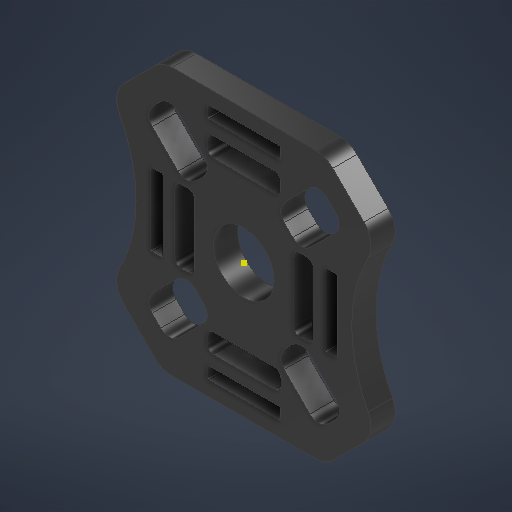
# Autodesk Inventor part: atasandrone
Saved by Autodesk Inventor 2026.1 (Build 301233000, 233)
## iProperties
Created: 2026-03-03
Part Number: atasandrone
Material: Generic
Document SubType Name: Modeling
Designer: ayjuni03
Density: 1 g/cm^3
Appearance: Default
Author: ayjuni03
Autodesk Inventor part; units mm, degrees
ref_plane "YZ Plane" through (0, 0, 0) normal (1, 0, 0) x (0, 1, 0)
ref_plane "XZ Plane" through (0, 0, 0) normal (0, 1, 0) x (-1, 0, 0)
ref_plane "XY Plane" through (0, 0, 0) normal (0, 0, 1) x (1, 0, 0)
sketch "Sketch1" plane through (0, 0, 0) normal (0, 0, 1) x (1, 0, 0)
  line L0 (0, 0) -> (55, 0)
  line L1 (55, 0) -> (-55, 0)
  line L2 (-55, 0) -> (-55, 55)
  line L3 (-55, 33.743) -> (-55, -33.7433)
  line L4 (-29.6762, -55) -> (29.5764, -55)
  line L5 (-29.5258, 55) -> (29.5764, 55)
  line L6 (55.0505, 33.743) -> (55.0505, -33.7433)
  line L7 (-49.4757, -39.2903) -> (-36.7617, -52.0566) construction
  line L8 (-49.4757, -39.2903) -> (-36.7617, -52.0566)
  line L9 (-55, -33.7433) -> (55.0505, -33.7433) construction
  line L10 (-55, -55) -> (-33.8303, -55) construction
  line L11 (55.0505, -55) -> (33.7065, -55) construction
  line L12 (36.633, -52.0856) -> (49.4815, -39.2896)
  line L13 (-55, -55) -> (-55, -33.7433) construction
  line L14 (-55, -55) -> (-55, -33.7433) construction
  line L15 (-55, -33.7433) -> (-55, -55) construction
  line L16 (-55, -33.7433) -> (-55, -55) construction
  line L17 (-55, 55) -> (-55, 33.743) construction
  line L18 (-55, 55) -> (-33.656, 55) construction
  line L19 (-36.5824, 52.0855) -> (-49.4311, 39.2892)
  line L20 (55.0505, 55) -> (47.34, 55) construction
  line L21 (33.7065, 55) -> (55.0505, 55) construction
  line L22 (55.0505, 55) -> (55.0505, 33.743) construction
  line L23 (49.4816, 39.2892) -> (36.633, 52.0855)
  arc A0 (-51.2319, -27.5622) -> (-51.2185, 27.5365) centre (-103.3983, -0.0002) ccw
  arc A1 (51.2691, 27.5365) -> (51.269, -27.5368) centre (103.4489, -0.0002) ccw
  arc A2 (-49.4311, 39.2892) -> (-51.2185, 27.5365) centre (-42.3745, 32.2037) ccw
  arc A3 (-29.5258, 55) -> (-36.5824, 52.0855) centre (-29.5258, 45) ccw
  arc A4 (36.633, 52.0855) -> (29.5764, 55) centre (29.5764, 45) ccw
  arc A5 (51.2691, 27.5365) -> (49.4816, 39.2892) centre (42.425, 32.2037) ccw
  arc A6 (49.4815, -39.2896) -> (51.269, -27.5368) centre (42.425, -32.204) ccw
  arc A7 (29.5764, -55) -> (36.633, -52.0856) centre (29.5764, -45) ccw
  arc A8 (-36.7617, -52.0566) -> (-29.6762, -55) centre (-29.6762, -45) ccw
  arc A9 (-51.2319, -27.5622) -> (-49.4757, -39.2903) centre (-42.3902, -32.2338) ccw
  line L24 (-0.0499, -55) -> (-0.0499, -49) construction
  line L25 (-0.0499, -49) -> (14.4501, -49)
  line L26 (14.9501, -49) -> (-14.5499, -49)
  line L27 (-15.0499, -48.5) -> (-15.0499, -44.5)
  line L28 (-14.5499, -44) -> (14.4501, -44)
  line L29 (14.9501, -44.5) -> (14.9501, -48.5)
  arc A10 (14.4501, -49) -> (14.9501, -48.5) centre (14.4501, -48.5) ccw
  arc A11 (14.9501, -44.5) -> (14.4501, -44) centre (14.4501, -44.5) ccw
  arc A12 (-14.5499, -44) -> (-15.0499, -44.5) centre (-14.5499, -44.5) ccw
  arc A13 (-15.0499, -48.5) -> (-14.5499, -49) centre (-14.5499, -48.5) ccw
  line L30 (-36.0332, -38.6169) -> (-43.1187, -45.6734) construction
  line L31 (-36.0332, -38.6169) -> (-34.269, -40.3883) construction
  line L32 (-34.269, -40.3883) -> (-37.7973, -36.8455) construction
  line L33 (-37.7828, -29.7744) -> (-27.1545, -19.1896) construction
  line L34 (-20.0834, -19.2041) -> (-16.5552, -22.7469) construction
  line L35 (-16.5697, -29.8179) -> (-27.198, -40.4028) construction
  line L36 (-16.5697, -29.8179) -> (-27.198, -40.4028)
  line L37 (-37.7828, -29.7744) -> (-23.6117, -15.6613)
  line L38 (-16.5552, -22.7469) -> (-20.0834, -19.2041)
  arc A14 (-37.7828, -29.7744) -> (-37.7973, -36.8455) centre (-34.2545, -33.3172) ccw
  arc A15 (-34.269, -40.3883) -> (-27.198, -40.4028) centre (-30.7263, -36.86) ccw
  arc A16 (-16.5697, -29.8179) -> (-16.5552, -22.7469) centre (-20.0979, -26.2752) ccw
  arc A17 (-20.0834, -19.2041) -> (-27.1545, -19.1896) centre (-23.6262, -22.7324) ccw
  line L39 (-41.3256, -33.3027) -> (-40.8868, -33.7433)
  line L40 (-37.7973, -36.8455) -> (-34.269, -40.3883)
  line L41 (-42.3902, -32.2338) -> (-34.269, -40.3883) construction
  line L42 (-30.7408, -43.931) -> (-29.6762, -45) construction
  line L43 (-43.1187, -45.6734) -> (43.0572, -45.6876) construction
  line L44 (43.0572, -45.6876) -> (36.0007, -38.602) construction
  line L45 (36.0007, -38.602) -> (37.7721, -36.8379) construction
  line L46 (27.1583, -40.3516) -> (16.5734, -29.7233) construction
  line L47 (13.0451, -26.1805) -> (20.1307, -19.124) construction
  line L48 (27.2017, -19.1385) -> (37.7866, -29.7668) construction
  line L49 (20.1307, -19.124) -> (16.5879, -22.6523)
  line L50 (27.1583, -40.3516) -> (16.5734, -29.7233)
  line L51 (27.2017, -19.1385) -> (37.7866, -29.7668)
  arc A18 (27.2017, -19.1385) -> (20.1307, -19.124) centre (23.659, -22.6668) ccw
  arc A19 (16.5879, -22.6523) -> (16.5734, -29.7233) centre (20.1162, -26.195) ccw
  arc A20 (37.7721, -36.8379) -> (37.7866, -29.7668) centre (34.2438, -33.2951) ccw
  line L52 (41.3149, -33.3096) -> (40.8793, -33.7433) construction
  line L53 (37.7721, -36.8379) -> (34.2293, -40.3661) construction
  line L54 (30.6865, -43.8944) -> (37.7721, -36.8379) construction
  line L55 (40.8793, -33.7433) -> (41.3149, -33.3096) construction
  line L56 (42.425, -32.204) -> (40.8793, -33.7433) construction
  line L57 (37.7721, -36.8379) -> (29.5764, -45) construction
  line L58 (41.3149, -33.3096) -> (40.8793, -33.7433)
  line L59 (37.7721, -36.8379) -> (34.2293, -40.3661)
  arc A21 (27.1583, -40.3516) -> (34.2293, -40.3661) centre (30.701, -36.8234) ccw
  circle A22 centre (0, 0) radius 12.5
  line L60 (-0.0499, -44) -> (-0.0499, -39) construction
  line L61 (-0.0499, -39) -> (12.6162, -39) construction
  line L62 (12.6162, -39) -> (-0.0499, -39)
  line L63 (-0.0499, -39) -> (-12.5979, -39)
  line L64 (-15.0979, -36.5) -> (-15.0979, -33.5)
  line L65 (-12.5979, -31) -> (12.6162, -31)
  line L66 (15.1162, -33.5) -> (15.1162, -36.5)
  arc A23 (15.1162, -33.5) -> (12.6162, -31) centre (12.6162, -33.5) ccw
  arc A24 (12.6162, -39) -> (15.1162, -36.5) centre (12.6162, -36.5) ccw
  arc A25 (-12.5979, -31) -> (-15.0979, -33.5) centre (-12.5979, -33.5) ccw
  arc A26 (-15.0979, -36.5) -> (-12.5979, -39) centre (-12.5979, -36.5) ccw
  line L67 (-44.3983, -0.0145) -> (-38.3983, 0) construction
  line L68 (44.4489, -0.0001) -> (38.4489, 0) construction
  line L69 (-38.3983, 0) -> (-38.3983, 14.5)
  line L70 (-38.3983, 15) -> (-38.3983, -14.5)
  line L71 (-37.8983, -15) -> (-33.8983, -15)
  line L72 (-33.3983, -14.5) -> (-33.3983, 14.5)
  line L73 (-33.8983, 15) -> (-37.8983, 15)
  arc A27 (-33.3983, 14.5) -> (-33.8983, 15) centre (-33.8983, 14.5) ccw
  arc A28 (-37.8983, 15) -> (-38.3983, 14.5) centre (-37.8983, 14.5) ccw
  arc A29 (-38.3983, -14.5) -> (-37.8983, -15) centre (-37.8983, -14.5) ccw
  arc A30 (-33.8983, -15) -> (-33.3983, -14.5) centre (-33.8983, -14.5) ccw
  line L74 (-33.3983, 0) -> (-28.3983, 0) construction
  line L75 (-28.3983, 0) -> (-28.3983, 12.5)
  line L76 (-28.3983, 12.5) -> (-28.3983, -12.5)
  line L77 (-25.8983, -15) -> (-22.8983, -15)
  line L78 (-20.3983, -12.5) -> (-20.3983, 12.5)
  line L79 (-22.8983, 15) -> (-25.8983, 15)
  arc A31 (-20.3983, 12.5) -> (-22.8983, 15) centre (-22.8983, 12.5) ccw
  arc A32 (-25.8983, 15) -> (-28.3983, 12.5) centre (-25.8983, 12.5) ccw
  arc A33 (-28.3983, -12.5) -> (-25.8983, -15) centre (-25.8983, -12.5) ccw
  arc A34 (-22.8983, -15) -> (-20.3983, -12.5) centre (-22.8983, -12.5) ccw
  line L80 (38.4489, 0) -> (38.4489, -14.5)
  line L81 (38.4489, -15) -> (38.4489, 14.5)
  line L82 (37.9489, 15) -> (33.9489, 15)
  line L83 (33.4489, 14.5) -> (33.4489, -14.5)
  line L84 (33.9489, -15) -> (37.9489, -15)
  arc A35 (38.4489, 14.5) -> (37.9489, 15) centre (37.9489, 14.5) ccw
  arc A36 (33.9489, 15) -> (33.4489, 14.5) centre (33.9489, 14.5) ccw
  arc A37 (33.4489, -14.5) -> (33.9489, -15) centre (33.9489, -14.5) ccw
  arc A38 (37.9489, -15) -> (38.4489, -14.5) centre (37.9489, -14.5) ccw
  line L85 (33.4489, 0) -> (28.4489, 0) construction
  line L86 (28.4489, 0) -> (28.4489, 12.5)
  line L87 (28.4489, 15) -> (28.4489, -12.5)
  line L88 (25.9489, -15) -> (22.9489, -15)
  line L89 (20.4489, -12.5) -> (20.4489, 12.5)
  line L90 (22.9489, 15) -> (25.9489, 15)
  arc A39 (28.4489, 12.5) -> (25.9489, 15) centre (25.9489, 12.5) ccw
  arc A40 (22.9489, 15) -> (20.4489, 12.5) centre (22.9489, 12.5) ccw
  arc A41 (20.4489, -12.5) -> (22.9489, -15) centre (22.9489, -12.5) ccw
  arc A42 (25.9489, -15) -> (28.4489, -12.5) centre (25.9489, -12.5) ccw
  line L91 (0.0253, 55) -> (0.0253, 49) construction
  line L92 (0.0253, 49) -> (14.5253, 49)
  line L93 (15.0253, 49) -> (-14.4747, 49)
  line L94 (-14.9747, 48.5) -> (-14.9747, 44.5)
  line L95 (-14.4747, 44) -> (14.5253, 44)
  line L96 (15.0253, 44.5) -> (15.0253, 48.5)
  arc A43 (15.0253, 48.5) -> (14.5253, 49) centre (14.5253, 48.5) ccw
  arc A44 (14.5253, 44) -> (15.0253, 44.5) centre (14.5253, 44.5) ccw
  arc A45 (-14.9747, 44.5) -> (-14.4747, 44) centre (-14.4747, 44.5) ccw
  arc A46 (-14.4747, 49) -> (-14.9747, 48.5) centre (-14.4747, 48.5) ccw
  line L97 (0.0253, 44) -> (0.0253, 39) construction
  line L98 (0.0253, 39) -> (12.5253, 39)
  line L99 (15.0253, 36.5) -> (15.0253, 33.5)
  line L100 (12.5253, 31) -> (-12.4747, 31)
  line L101 (-14.9747, 33.5) -> (-14.9747, 36.5)
  line L102 (-12.4747, 39) -> (0.0253, 39)
  arc A47 (-12.4747, 39) -> (-14.9747, 36.5) centre (-12.4747, 36.5) ccw
  arc A48 (-14.9747, 33.5) -> (-12.4747, 31) centre (-12.4747, 33.5) ccw
  arc A49 (12.5253, 31) -> (15.0253, 33.5) centre (12.5253, 33.5) ccw
  arc A50 (15.0253, 36.5) -> (12.5253, 39) centre (12.5253, 36.5) ccw
  line L103 (29.5764, 45) -> (37.7721, 36.8377) construction
  line L104 (37.7721, 36.8377) -> (36.0007, 38.6019) construction
  line L105 (36.0007, 38.6019) -> (43.0573, 45.6873) construction
  line L106 (36.0007, 38.6019) -> (37.7721, 36.8377)
  line L107 (41.3148, 33.3094) -> (34.2293, 40.366)
  line L108 (27.1583, 40.3516) -> (16.5733, 29.7233)
  line L109 (37.7865, 29.7666) -> (27.2016, 19.1384)
  line L110 (20.1305, 19.124) -> (16.5878, 22.6523)
  arc A51 (37.7865, 29.7666) -> (37.7721, 36.8377) centre (34.2438, 33.295) ccw
  arc A52 (20.1305, 19.124) -> (27.2016, 19.1384) centre (23.6588, 22.6667) ccw
  arc A53 (16.5733, 29.7233) -> (16.5878, 22.6523) centre (20.1161, 26.195) ccw
  arc A54 (34.2293, 40.366) -> (27.1583, 40.3516) centre (30.701, 36.8233) ccw
  line L111 (-42.3745, 32.2037) -> (-29.5258, 45) construction
  line L112 (-29.5258, 45) -> (-35.9502, 38.6019) construction
  line L113 (-43.0068, 45.6873) -> (-35.9502, 38.6019) construction
  line L114 (-35.9502, 38.6019) -> (-34.1788, 40.366)
  line L115 (-30.636, 43.8943) -> (-37.7215, 36.8377)
  line L116 (-37.736, 29.7666) -> (-27.151, 19.1384)
  line L117 (-20.08, 19.124) -> (-16.5372, 22.6523)
  line L118 (-16.5228, 29.7233) -> (-27.1077, 40.3516)
  arc A55 (-27.1077, 40.3516) -> (-34.1788, 40.366) centre (-30.6505, 36.8233) ccw
  arc A56 (-37.7215, 36.8377) -> (-37.736, 29.7666) centre (-34.1932, 33.295) ccw
  arc A57 (-27.151, 19.1384) -> (-20.08, 19.124) centre (-23.6083, 22.6667) ccw
  arc A58 (-16.5372, 22.6523) -> (-16.5228, 29.7233) centre (-20.0656, 26.195) ccw
  point P0 (-15.0499, -49)
  point P1 (-15.0499, -44)
  point P2 (-15.0979, -39)
  point P3 (-15.0979, -31)
  point P4 (-38.3983, -15)
  point P5 (-33.3983, -15)
  point P6 (-28.3983, -15)
  point P7 (-20.3983, -15)
  point P8 (38.4489, 15)
  point P9 (33.4489, 15)
  point P10 (28.4489, -15)
  point P11 (20.4489, -15)
  point P12 (-14.9747, 49)
  point P13 (-14.9747, 44)
  point P14 (15.0253, 39)
  point P15 (15.0253, 31)
  point P16 (-14.9747, 31)
  point P17 (-14.9747, 39)
  point P18 (30.6866, 43.8943)
  point P19 (13.045, 26.1806)
  point P20 (-41.2643, 33.3094)
  point P21 (-23.6227, 15.5957)
  dimension "d0" = 55
  dimension "d1" = 110
  dimension "d2" = 55
  dimension "d3" = 110
  dimension "d4" = 30
  dimension "d5" = 21.344
  dimension "d6" = 21.257
  dimension "d7" = 21.344
  dimension "d8" = 21.344
  dimension "d9" = 21.257
  dimension "d10" = 59
  dimension "d11" = 59
  dimension "d12" = 10
  dimension "d13" = 6
  dimension "d14" = 15
  dimension "d15" = 30
  dimension "d16" = 5
  dimension "d17" = 0.5
  dimension "d18" = 7.5
  dimension "d19" = 15
  dimension "d20" = 25
  dimension "d21" = 5
  dimension "d22" = 7.5
  dimension "d23" = 15
  dimension "d24" = 25
  dimension "d25" = 5
  dimension "d26" = 5
  dimension "d27" = 25
  dimension "d28" = 5
  dimension "d29" = 8
  dimension "d30" = 2.5
  dimension "d31" = 6
  dimension "d32" = 6
  dimension "d33" = 15
  dimension "d34" = 30
  dimension "d35" = 5
  dimension "d36" = 0.5
  dimension "d37" = 5
  dimension "d38" = 8
  dimension "d39" = 2.5
  dimension "d40" = 15
  dimension "d41" = 30
  dimension "d42" = 5
  dimension "d43" = 0.5
  dimension "d44" = 5
  dimension "d45" = 8
  dimension "d46" = 2.5
  dimension "d47" = 6
  dimension "d48" = 15
  dimension "d49" = 30
  dimension "d50" = 5
  dimension "d51" = 0.5
  dimension "d52" = 5
  dimension "d53" = 15
  dimension "d54" = 8
  dimension "d55" = 30
  dimension "d56" = 2.5
  dimension "d57" = 7.5
  dimension "d58" = 15
  dimension "d59" = 25
  dimension "d60" = 5
  dimension "d61" = 7.5
  dimension "d62" = 15
  dimension "d63" = 25
  constraints: 238 end point, 122 point on circle, 112 tangent, 109 point on line, 59 centre point, 52 perpendicular, 42 equal radius, 18 collinear, 11 midpoint, 7 vertical, 2 horizontal, 2 parallel, 1 coincident
  measures "d0" distance of L0.start L0.end
  measures "d1" distance of L0.end L1.end
  measures "d2" distance of L1.end L2.end
  measures "d3" distance of L2.end L10.start
  measures "d4" distance of L3.end L10.end
  measures "d5" distance of L11.end L11.start
  measures "d6" distance of L3.start L2.end
  measures "d7" distance of L18.end L2.end
  measures "d8" distance of L21.start L20.start
  measures "d9" distance of L6.start L20.start
  measures "d10" radius of A0
  measures "d11" radius of A1
  measures "d12" radius of A2
  measures "d13" distance of L24.start L24.end
  measures "d14" distance of L24.end L26.start
  measures "d15" distance of L26.start point (-15.05, -49)
  measures "d16" distance of point (-15.05, -49) point (-15.05, -44)
  measures "d17" radius of A10
  measures "d18" distance of L30.start L42.start
  measures "d19" distance of L42.start L39.start
  measures "d20" distance of L39.start L37.end
  measures "d21" radius of A14
  measures "d22" distance of L44.end L52.start
  measures "d23" distance of L52.start L54.start
  measures "d24" distance of L54.start L47.start
  measures "d25" radius of A18
  measures "d26" radius of A21
  measures "d27" diameter of A22
  measures "d28" distance of L60.start L60.end
  measures "d29" distance of point (-15.098, -39) point (-15.098, -31)
  measures "d30" radius of A23
  measures "d31" distance of L67.start L67.end
  measures "d32" distance of L68.start L68.end
  measures "d33" distance of L67.end L70.start
  measures "d34" distance of L70.start point (-38.398, -15)
  measures "d35" distance of point (-38.398, -15) point (-33.398, -15)
  measures "d36" radius of A27
  measures "d37" distance of L74.start L74.end
  measures "d38" distance of point (-28.398, -15) point (-20.398, -15)
  measures "d39" radius of A31
  measures "d40" distance of L68.end L81.start
  measures "d41" distance of L81.start point (38.449, 15)
  measures "d42" distance of point (38.449, 15) point (33.449, 15)
  measures "d43" radius of A35
  measures "d44" distance of L85.start L85.end
  measures "d45" distance of point (28.449, -15) point (20.449, -15)
  measures "d46" radius of A39
  measures "d47" distance of L91.start L91.end
  measures "d48" distance of L91.end L93.start
  measures "d49" distance of L93.start point (-14.975, 49)
  measures "d50" distance of point (-14.975, 49) point (-14.975, 44)
  measures "d51" radius of A43
  measures "d52" distance of L97.start L97.end
  measures "d53" distance of L97.end point (15.025, 39)
  measures "d54" distance of point (15.025, 39) point (15.025, 31)
  measures "d55" distance of point (15.025, 31) point (-14.975, 31)
  measures "d56" radius of A47
  measures "d57" distance of L104.end L107.start
  measures "d58" distance of L107.start point (30.687, 43.894)
  measures "d59" distance of point (30.687, 43.894) point (13.045, 26.181)
  measures "d60" radius of A51
  measures "d61" distance of L112.end L115.start
  measures "d62" distance of L115.start point (-41.264, 33.309)
  measures "d63" distance of point (-41.264, 33.309) point (-23.623, 15.596)
extrude "Extrusion1" add sketch "Sketch1" along normal blind 10 contours A22 L1 L78 A31 L79 A32 L75 L72 A27 L73 A28 L69 A0 A2 L19 A3 L5 A4 L23 A5 A1 L0 L81 A35 L82 A36 L83 L86 A39 L90 A40 L89 | L0 L89 A41 L88 A42 L87 L83 A37 L84 A38 L80 A1 A6 L12 A7 L4 A8 L8 A9 A0 L1 L70 A29 L71 A30 L72 L76 A33 L77 A34 L78 A22
sketch "Sketch2" plane through (0, 0, 10) normal (0, 0, 1) x (1, 0, 0)
  point P0 (0, 0)
sketch "Sketch3" plane through (0, 0, 10) normal (0, 0, 1) x (1, 0, 0)
  point P0 (0, 0)
body "Solid1"
